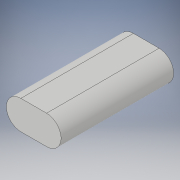
# Autodesk Inventor part: battery
Saved by Autodesk Inventor 2019 (Build 230136000, 136)
## iProperties
Created: 2019-06-25
Part Number: battery
Material: Generic
Document SubType Name: Modeling
Designer: Daniel
Density: 1 g/cm^3
Appearance: Default
Author: Daniel
Autodesk Inventor part; units mm, degrees
ref_plane "YZ Plane" through (0, 0, 0) normal (1, 0, 0) x (0, 1, 0)
ref_plane "XZ Plane" through (0, 0, 0) normal (0, 1, 0) x (-1, 0, 0)
ref_plane "XY Plane" through (0, 0, 0) normal (0, 0, 1) x (1, 0, 0)
sketch "Sketch1" plane through (0, 0, 0) normal (0, 0, 1) x (1, 0, 0)
  line L0 (0, 0) -> (20.32, 0) construction
  line L1 (0, -11.43) -> (20.32, -11.43)
  line L2 (20.32, 11.43) -> (0, 11.43)
  arc A0 (0, 11.43) -> (0, -11.43) centre (0, 0) ccw
  arc A1 (20.32, -11.43) -> (20.32, 11.43) centre (20.32, 0) ccw
  point P0 (10.16, 0)
  dimension "d0" = 22.86
  dimension "d2" = 43.18
  constraints: 8 end point, 4 point on circle, 4 tangent, 2 centre point, 1 horizontal, 1 midpoint, 1 parallel
  measures "d0" distance between parallel lines of L1 L2
extrude "Extrusion1" add sketch "Sketch1" along normal blind 88.9
body "Solid1"
